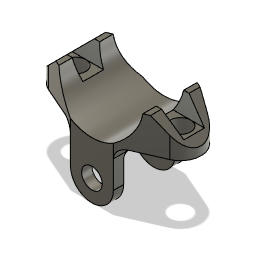
0.883.3554 - Demi-bride à chape pour bras de rappel sur tube 49 - VZC 21465_203526 (Autodesk Fusion 360 design; units mm, degrees)
Autodesk Fusion 360 part; units mm, degrees
sketch "Sketch1" plane through (0, 0, 0) normal (0, 0, 1) x (1, 0, 0)
  line L0 (0, 0) -> (100, 0) construction
  line L1 (0, 0) -> (-100, 0) construction
  line L2 (0, -3) -> (100, -3) construction
  line L3 (0, -3) -> (-100, -3) construction
  circle A0 centre (0, 0) radius 24.6 construction
  circle A1 centre (0, 0) radius 28.5 construction
  line L4 (0, -23) -> (100, -23) construction
  line L5 (0, -23) -> (-100, -23) construction
  line L6 (0, 0) -> (0, -150) construction
  line L7 (0, 0) -> (0, 150) construction
  line L8 (-30.5, 0) -> (-30.5, -150) construction
  line L9 (-30.5, 0) -> (-30.5, 150) construction
  line L10 (30.5, 0) -> (30.5, 150) construction
  line L11 (30.5, 0) -> (30.5, -150) construction
  line L12 (-30.5, -23) -> (-42.5, -23)
  line L13 (-42.5, -23) -> (-42.5, -18)
  line L14 (-42.5, -18) -> (-12.5, -18) construction
  line L15 (-42.5, -18) -> (-27.5, -3)
  line L16 (-24.5998, -0.0998) -> (-24.5, 0)
  line L17 (-24.4164, -3) -> (-27.5, -3)
  line L18 (24.4164, -3) -> (27.5, -3)
  line L19 (42.5, -18) -> (27.5, -3)
  line L20 (30.5, -23) -> (42.5, -23)
  line L21 (42.5, -23) -> (42.5, -18)
  arc A2 (-24.4164, -3) -> (24.4164, -3) centre (0, 0) ccw
  line L22 (0, -45) -> (-100, -45) construction
  line L23 (0, -45) -> (100, -45) construction
  circle A3 centre (0, -45) radius 6
  circle A4 centre (0, -45) radius 12.5 construction
  line L24 (-12.5, -45) -> (-12.5, -29)
  line L25 (-30.5, -23) -> (-18.5, -23)
  line L26 (12.5, -45) -> (12.5, -29)
  line L27 (30.5, -23) -> (18.5, -23)
  arc A5 (-12.5, -45) -> (12.5, -45) centre (0, -45) ccw
  arc A6 (-12.5, -29) -> (-18.5, -23) centre (-18.5, -29) ccw
  arc A7 (18.5, -23) -> (12.5, -29) centre (18.5, -29) ccw
  dimension "d4" = 3
  dimension "d5" = 49.2
  dimension "d6" = 57
  dimension "d7" = 23
  dimension "d10" = 30.5
  dimension "d11" = 30.5
  dimension "d12" = 12
  dimension "d13" = 5
  dimension "d14" = 45
  dimension "d16" = 24.6
  dimension "d17" = 45
  dimension "d18" = 12
  dimension "d19" = 25
  dimension "d20" = 6
  dimension "d21" = 6
  constraint coincident L0.start L1.start
  constraint horizontal L0
  constraint horizontal L1
  constraint concentric A0 A1
  constraint vertical L6
  constraint vertical L7
  constraint coincident L8 L12.start
  constraint coincident L5 L12.start
  constraint horizontal L14
  constraint coincident L3 L15.end
  constraint coincident A0 L16.start
  constraint collinear L15 L16
  constraint coincident L1 L16.end
  constraint coincident A0 L17.start
  constraint coincident L3 L17.start
  constraint parallel L3 L17
  constraint horizontal L12
  constraint symmetric L6 L12.start L20.start
  constraint symmetric L6 L12.end L20.end
  constraint symmetric L6 L13.end L19.start
  constraint symmetric L6 L15.end L18.end
  constraint symmetric L6 L17.start L18.start
  constraint coincident L22.start L23.start
  constraint concentric A3 A4
  constraint coincident A4 L24.start
  constraint coincident L22 L24.start
  constraint tangent A4 L24
  constraint perpendicular L5 L24
  constraint symmetric L6 L24.start L26.start
  constraint tangent L26 A5
  constraint tangent L24 A6
  constraint tangent L25 A6
  constraint tangent L26 A7
  constraint tangent L27 A7
  constraint vertical L26
  constraint horizontal L27
  constraint vertical L21
  measures "d5" diameter of A0
  measures "d6" diameter of A1
  measures "d12" distance of L12.start L12.end
  measures "d13" distance of L12.end L13.end
  measures "d14" angle of L14 L15
  measures "d16" radius of A2
  measures "d18" diameter of A3
  measures "d19" diameter of A4
  measures "d20" radius of A6
  measures "d21" radius of A7
extrude "Extrude1" add sketch "Sketch1" along normal mid plane 42
sketch "Sketch2" plane through (0, 0, 0) normal (0, 1, 0) x (1, 0, 0)
  line L0 (-24.4164, 21) -> (24.4164, 21) construction
  line L1 (-27.5, 21) -> (-24.4164, 21) construction
  line L2 (-42.5, 21) -> (-27.5, 21) construction
  line L3 (24.4164, 21) -> (27.5, 21) construction
  line L4 (27.5, 21) -> (42.5, 21) construction
  line L5 (6, -21) -> (-6, -21) construction
  line L6 (18.5, -21) -> (42.5, -21) construction
  line L7 (42.5, -21) -> (27.5, -21) construction
  line L8 (27.5, -21) -> (24.4164, -21) construction
  line L9 (24.4164, -21) -> (-24.4164, -21) construction
  line L10 (-24.4164, -21) -> (-27.5, -21) construction
  line L11 (-27.5, -21) -> (-42.5, -21) construction
  line L12 (-42.5, -21) -> (-18.5, -21) construction
  line L13 (-12.5, -21) -> (-18.5, -21) construction
  line L14 (-12.5, -21) -> (12.5, -21) construction
  line L15 (18.5, -21) -> (12.5, -21) construction
  line L16 (42.5, 21) -> (42.5, -21) construction
  line L17 (42.5, -21) -> (42.5, 21) construction
  line L18 (-42.5, 21) -> (-42.5, -21) construction
  line L19 (-42.5, -21) -> (-42.5, 21) construction
  circle A0 centre (-30.5, 0) radius 12 construction
  circle A1 centre (30.5, 0) radius 12 construction
  line L20 (0, 21) -> (0, -21) construction
  line L21 (-12.5, 21) -> (-12.5, -21) construction
  line L22 (12.5, 21) -> (12.5, -21) construction
  line L23 (-12.5, 21) -> (12.5, 21)
  line L24 (-12.5, -21) -> (12.5, -21)
  line L25 (12.5, -21) -> (35.3207, -10.9891)
  line L26 (12.5, 21) -> (35.3207, 10.9891)
  line L27 (-12.5, 21) -> (-35.3207, 10.9891)
  line L28 (-12.5, -21) -> (-35.3207, -10.9891)
  arc A2 (35.3207, -10.9891) -> (35.3207, 10.9891) centre (30.5, 0) ccw
  arc A3 (-35.3207, 10.9891) -> (-35.3207, -10.9891) centre (-30.5, 0) ccw
  line L29 (12.5, 21) -> (42.5, 21)
  line L30 (12.5, -21) -> (42.5, -21)
  line L31 (42.5, -21) -> (42.5, 21)
  line L32 (-42.5, 21) -> (-12.5, 21)
  line L33 (-42.5, -21) -> (-12.5, -21)
  line L34 (-42.5, -21) -> (-42.5, 21)
  circle A4 centre (30.5, 0) radius 6
  circle A5 centre (-30.5, 0) radius 6
  dimension "d24" = 24
  dimension "d25" = 24
  dimension "d26" = 12.5
  dimension "d27" = 12.5
  dimension "d28" = 12
  dimension "d29" = 12
  constraint midpoint L0 L20.start
  constraint midpoint L14 L20.end
  constraint perpendicular L22 L23
  constraint perpendicular L22 L24
  constraint coincident A1 L25.end
  constraint tangent A1 L25
  constraint coincident A1 L26.end
  constraint tangent A1 L26
  constraint coincident A0 L27.end
  constraint tangent A0 L27
  constraint parallel L25 L27
  constraint coincident A0 L28.end
  constraint tangent A0 L28
  constraint parallel L26 L28
  constraint tangent L17 A2
  constraint tangent L19 A3
  constraint coincident L4.end L16.start
  constraint perpendicular L16 L29
  constraint coincident L6.end L7.start
  constraint perpendicular L16 L30
  constraint coincident L2.start L18.start
  constraint perpendicular L31 L32
  constraint coincident L11.end L12.start
  constraint coincident L13.start L14.start
  constraint concentric A1 A4
  constraint concentric A0 A5
  measures "d24" diameter of A0
  measures "d25" diameter of A1
  measures "d28" diameter of A4
  measures "d29" diameter of A5
extrude "Extrude2" cut sketch "Sketch2" against normal through all contours L27 A3 L32 L34 | L26 A2 L29 L31 | L28 A3 L33 L34 | L25 A2 L30 L31 | A4 | A5
sketch "Sketch3" plane through (0, 0, 0) normal (1, 0, 0) x (0, 0, -1)
  line L0 (-21, -51) -> (-21, -39) construction
  line L1 (-21, -29) -> (-21, -21.1875) construction
  line L2 (-21, -24.6) -> (-21, -21.1875) construction
  line L3 (-21, -21.1875) -> (-21, -29) construction
  line L4 (-21, -29) -> (-21, -45) construction
  line L5 (-21, -45) -> (-21, -57.5) construction
  line L6 (-21, -45) -> (-21, -29) construction
  line L7 (21, -21.1875) -> (21, -29) construction
  line L8 (21, -29) -> (21, -45) construction
  line L9 (21, -57.5) -> (21, -45) construction
  line L10 (21, -45) -> (21, -29) construction
  line L11 (21, -29) -> (21, -21.1875) construction
  line L12 (21, -21.1875) -> (21, -24.6) construction
  line L13 (21, -39) -> (21, -51) construction
  line L14 (21, -45) -> (-21, -45) construction
  line L15 (-21, -45) -> (-21, -57.5) construction
  line L16 (-21, -45) -> (21, -45) construction
  line L17 (21, -57.5) -> (21, -45) construction
  line L18 (21, -45) -> (-21, -45) construction
  line L19 (-21, -45) -> (-21, -29) construction
  line L20 (-21, -29) -> (21, -29) construction
  line L21 (21, -29) -> (21, -45) construction
  line L22 (-5.1962, -3) -> (-14.4199, -3) construction
  line L23 (14.4199, -3) -> (5.1962, -3) construction
  line L24 (-5.1962, -3) -> (5.1962, -3) construction
  arc A0 (-5.1962, -3) -> (5.1962, -3) centre (0, -6) ccw construction
  line L25 (-5.1962, -3) -> (5.1962, -3) construction
  line L26 (6, -23) -> (-6, -23) construction
  line L27 (0, 0) -> (0, -75) construction
  line L28 (-6, 0) -> (-6, -75) construction
  line L29 (-8, 0) -> (-8, -75) construction
  line L30 (6, 0) -> (6, -75) construction
  line L31 (8, 0) -> (8, -75) construction
  line L32 (21, -57.5) -> (-21, -57.5) construction
  line L33 (21, -57.5) -> (15, -57.5)
  line L34 (-21, -57.5) -> (-15, -57.5)
  line L35 (0, 0) -> (40, 0) construction
  line L36 (0, 0) -> (-40, 0) construction
  line L37 (0, -28.5) -> (-40, -28.5) construction
  line L38 (15, -57.5) -> (15, -32)
  line L39 (-15, -57.5) -> (-15, -32)
  line L40 (-12, -29) -> (12, -29)
  line L41 (15, -57.5) -> (-15, -57.5)
  arc A1 (15, -32) -> (12, -29) centre (12, -32) ccw
  arc A2 (-12, -29) -> (-15, -32) centre (-12, -32) ccw
  line L42 (0, -3) -> (-8, -3)
  line L43 (0, -3) -> (8, -3)
  line L44 (14.4199, -14) -> (5.1962, -14) construction
  line L45 (-5.1962, -14) -> (5.1962, -14) construction
  line L46 (-5.1962, -14) -> (-14.4199, -14) construction
  line L47 (6, -14) -> (8, -3)
  line L48 (-6, -14) -> (-8, -3)
  line L49 (-6, -14) -> (6, -14)
  point P0 (-15.7726, -3)
  point P1 (15.7726, -3)
  point P2 (21, -21.1875)
  point P3 (-21, -21.1875)
  dimension "d32" = 6
  dimension "d33" = 8
  dimension "d34" = 6
  dimension "d35" = 8
  dimension "d36" = 6
  dimension "d37" = 6
  dimension "d41" = 3
  dimension "d42" = 3
  dimension "d43" = 8
  dimension "d44" = 11
  constraint coincident L27.start L35.start
  constraint vertical L27
  constraint coincident L9.start L17.start
  constraint coincident L5.end L15.end
  constraint horizontal L34
  constraint horizontal L33
  constraint horizontal L36
  constraint horizontal L35
  constraint perpendicular L20 L38
  constraint parallel L36 L37
  constraint perpendicular L20 L39
  constraint tangent L38 A1
  constraint tangent L40 A1
  constraint tangent L39 A2
  constraint tangent L40 A2
  constraint horizontal L40
  constraint midpoint L25 L42.start
  constraint coincident L23 L43.end
  constraint coincident L31 L43.end
  constraint perpendicular L31 L43
  constraint coincident L44 L47.start
  constraint coincident L30 L47.start
  constraint coincident L46 L48.start
  constraint coincident L28 L48.start
  constraint perpendicular L30 L49
  constraint horizontal L42
  measures "d36" distance of L9.start L33.end
  measures "d37" distance of L5.end L34.end
  measures "d41" radius of A1
  measures "d42" radius of A2
  measures "d43" distance of L42.start L42.end
extrude "Extrude3" cut sketch "Sketch3" along normal through all and the other way through all
equation "d5 = ( 24.6 * 2 ) * 1 mm"
equation "d6 = ( 28.5 * 2 ) * 1 mm"
